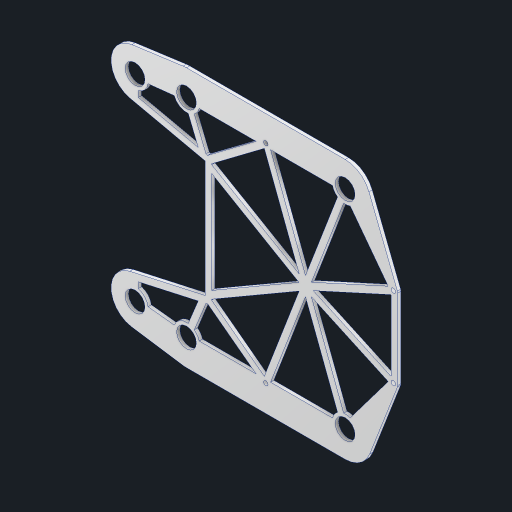
# Autodesk Inventor part: OUTK_002_ShotPlateNoReceptacle
Saved by Autodesk Inventor 2024.2 (Build 282272000, 272)
## iProperties
Created: 2024-11-24
Part Number: OUTK_002_ShotPlateNoReceptacle
Material: Aluminum 6061
Document SubType Name: Modeling
Designer: Bryan
Density: 2.7 g/cm^3
Appearance: Aluminum - Flat
Mass: 1558.28 g
Surface Area: 2532.23 cm^2
Volume: 577.142 cm^3
Author: Bryan
Autodesk Inventor part; units mm, degrees
ref_plane "YZ Plane" through (0, 0, 0) normal (1, 0, 0) x (0, 1, 0)
ref_plane "XZ Plane" through (0, 0, 0) normal (0, 1, 0) x (-1, 0, 0)
ref_plane "XY Plane" through (0, 0, 0) normal (0, 0, 1) x (1, 0, 0)
sketch "Sketch1" plane through (0, 0, 0) normal (0, 0, 1) x (1, 0, 0)
  circle A0 centre (0, 142.875) radius 63.5 construction
  circle A1 centre (0, 142.875) radius 25.4 construction
  circle A2 centre (0, -142.875) radius 25.4 construction
  circle A3 centre (0, -142.875) radius 63.5 construction
  line L0 (0, 79.375) -> (0, 79.375) construction
  line L1 (0, -79.375) -> (0, -79.375) construction
  line L2 (0, 0) -> (228.6, 0) construction
  line L3 (0, 142.875) -> (304.8, 142.875) construction
  line L4 (304.8, 142.875) -> (304.8, -142.875) construction
  line L5 (304.8, -142.875) -> (0, -142.875) construction
  circle A4 centre (228.6, 0) radius 127 construction
  circle A5 centre (0, 142.875) radius 14.2875
  circle A6 centre (0, -142.875) radius 14.2875
  circle A7 centre (0, 142.875) radius 34.925 construction
  circle A8 centre (0, -142.875) radius 34.925 construction
  circle A9 centre (74.585, -150.8125) radius 22.225 construction
  circle A10 centre (74.585, -150.8125) radius 33.3375 construction
  circle A11 centre (74.585, -150.8125) radius 11.1125 construction
  line L6 (74.585, -139.7) -> (74.585, -128.5875) construction
  line L7 (74.585, -117.475) -> (74.585, -128.5875) construction
  circle A12 centre (304.8, -150.8125) radius 33.3375 construction
  circle A13 centre (304.8, -150.8125) radius 14.2875
  circle A14 centre (374.65, 58.0572) radius 6.35 construction
  circle A15 centre (374.65, -58.0572) radius 6.35 construction
  line L8 (304.8, 150.8125) -> (374.65, 58.0572) construction
  line L9 (374.65, 58.0572) -> (374.65, -58.0572) construction
  line L10 (374.65, -58.0572) -> (304.8, -150.8125) construction
  line L11 (-118.745, 84.5312) -> (101.6, 84.5312) construction
  line L12 (101.6, 84.5312) -> (101.6, -84.5312) construction
  line L13 (101.6, -84.5312) -> (-118.745, -84.5312) construction
  line L14 (-118.745, -84.5312) -> (-118.745, 84.5312) construction
  line L15 (0, 142.875) -> (0, 84.5312) construction
  line L16 (0, -84.5312) -> (0, -142.875) construction
  circle A16 centre (74.585, -150.8125) radius 14.2875
  line L17 (74.585, -117.475) -> (304.8, -117.475) construction
  circle A17 centre (74.585, 0) radius 127 construction
  circle A18 centre (0, 0) radius 127 construction
  circle A19 centre (0, 142.875) radius 6.35 construction
  circle A20 centre (74.585, 150.8125) radius 33.3375 construction
  circle A21 centre (304.8, 150.8125) radius 33.3375 construction
  circle A22 centre (304.8, 150.8125) radius 14.2875
  circle A23 centre (74.585, 150.8125) radius 14.2875
  circle A24 centre (74.585, 150.8125) radius 37.1475 construction
  circle A25 centre (304.8, 150.8125) radius 37.1475 construction
  circle A26 centre (304.8, -150.8125) radius 38.1 construction
  circle A27 centre (74.585, -150.8125) radius 38.1 construction
  line L18 (-4.7233, 177.4791) -> (69.5611, 187.6187)
  line L19 (74.585, 187.96) -> (304.8, 187.96)
  line L20 (339.3386, 164.488) -> (380.554, 60.3949)
  line L21 (381, 58.0572) -> (381, -58.0572)
  line L22 (68.953, -188.4939) -> (-5.1627, -177.4163)
  line L23 (220.4162, -245.7989) -> (237.7908, -293.5353) construction
  line L24 (237.7908, -293.5353) -> (381, -241.4114) construction
  line L25 (381, -241.4114) -> (363.6254, -193.675) construction
  line L26 (363.6254, -193.675) -> (220.4162, -245.7989) construction
  line L27 (-7.573, -108.7809) -> (101.6, -84.5312)
  line L28 (-7.573, 108.7809) -> (101.6, 84.5312)
  line L29 (101.6, 84.5312) -> (101.6, -84.5312)
  circle A28 centre (238.125, 0) radius 127
  line L30 (101.6, 0) -> (111.125, 0)
  line L31 (374.65, 0) -> (365.125, 0)
  circle A29 centre (220.4162, -245.7989) radius 3.2512 construction
  circle A30 centre (268.1526, -228.4242) radius 3.2512 construction
  circle A31 centre (315.889, -211.0496) radius 3.2512 construction
  circle A32 centre (363.6254, -193.675) radius 3.2512 construction
  circle A33 centre (237.7908, -293.5353) radius 3.2512 construction
  circle A34 centre (285.5272, -276.1606) radius 3.2512 construction
  circle A35 centre (333.2636, -258.786) radius 3.2512 construction
  circle A36 centre (381, -241.4114) radius 3.2512 construction
  line L32 (74.585, -188.9125) -> (304.8, -188.9125)
  line L33 (380.5737, -60.3445) -> (340.3424, -164.5364)
  arc A37 (-4.7233, 177.4791) -> (-7.573, 108.7809) centre (0, 142.875) ccw
  arc A38 (74.585, 187.96) -> (69.5611, 187.6187) centre (74.585, 150.8125) ccw
  arc A39 (339.3386, 164.488) -> (304.8, 187.96) centre (304.8, 150.8125) ccw
  arc A40 (381, 58.0572) -> (380.554, 60.3949) centre (374.65, 58.0572) ccw
  arc A41 (380.5737, -60.3445) -> (381, -58.0572) centre (374.65, -58.0572) ccw
  arc A42 (304.8, -188.9125) -> (340.3424, -164.5364) centre (304.8, -150.8125) ccw
  arc A43 (68.953, -188.4939) -> (74.585, -188.9125) centre (74.585, -150.8125) ccw
  arc A44 (-7.573, -108.7809) -> (-5.1627, -177.4163) centre (0, -142.875) ccw
  circle A45 centre (374.65, 58.0572) radius 3.2512
  circle A46 centre (374.65, -58.0572) radius 3.2512
  circle A47 centre (189.6925, 150.8125) radius 3.2512
  line L34 (74.585, 150.8125) -> (189.6925, 150.8125) construction
  line L35 (189.6925, 150.8125) -> (304.8, 150.8125) construction
  circle A48 centre (189.6925, -150.8125) radius 3.2512
  line L36 (74.585, -150.8125) -> (304.8, -150.8125) construction
  point P0 (0, 117.475)
  point P1 (0, -117.475)
  point P2 (304.8, 0)
  point P3 (228.6, -127)
  point P4 (228.6, -127)
  point P5 (355.6, 0)
  point P6 (0, 127)
  point P7 (0, 117.475)
  point P8 (0, 136.525)
  dimension "d1" = 50.8
  dimension "d16" = 44.45
  dimension "d20" = 22.225
  dimension "d33" = 12.7
  dimension "d0" = 127
  dimension "d3" = 285.75
  dimension "d4" = 254
  dimension "d6" = 158.75
  dimension "d7" = 234.95
  dimension "d11" = 28.575
  dimension "d12" = 28.575
  dimension "d13" = 69.85
  dimension "d14" = 69.85
  dimension "d19" = 76.2
  dimension "d22" = 304.8
  dimension "d24" = 28.575
  dimension "d26" = 12.7
  dimension "d27" = 12.7
  dimension "d28" = 19.05
  dimension "d29" = 220.345
  dimension "d30" = 169.0624
  dimension "d31" = 9.525
  dimension "d32" = 75.0062
  dimension "d34" = 9.525
  dimension "d35" = 19.05
  dimension "d37" = 3.81
  dimension "d38" = 3.81
  dimension "d39" = 4.7625
  dimension "d40" = 4.7625
  dimension "d43" = 20
  dimension "d44" = 6.5024
  dimension "d47" = 50.8
  dimension "d50" = 50.8
  dimension "d53" = 50.8
  dimension "d56" = 6.5024
  dimension "d57" = 6.5024
  dimension "d58" = 6.5024
  dimension "d105" = 230.215
  constraints: 74 end point, 41 centre point, 41 point on circle, 24 tangent, 21 coincident, 16 vertical alignment, 11 horizontal, 7 perpendicular, 7 point on line, 6 concentric, 6 equal length, 6 symmetric about line, 4 equal radius, 4 vertical, 3 horizontal alignment, 3 midpoint, 2 parallel, 41 other
  measures "d0" diameter of A0
  measures "d3" distance between parallel lines of L5 L3
  measures "d4" diameter of A4
  measures "d6" distance of L1.start L0.start
  measures "d7" distance of point (0, -117.475) point (0, 117.475)
  measures "d11" diameter of A5
  measures "d12" diameter of A6
  measures "d13" diameter of A7
  measures "d14" diameter of A8
  measures "d19" distance of point (304.8, 0) L2.end
  measures "d22" distance of L3.end A0.centre
  measures "d24" diameter of A13
  measures "d26" diameter of A14
  measures "d27" diameter of A15
  measures "d28" distance from line of L9 point (355.6, 0)
  measures "d29" distance of L12.end L13.end
  measures "d30" distance of L11.end L12.end
  measures "d31" distance from line of L17 A4.start
  measures "d32" distance of point (74.585, -150.812) point (0, -142.875)
  measures "d34" distance of point (0, 117.475) point (0, 127)
  measures "d35" distance of point (0, 117.475) point (0, 136.525)
  measures "d37" radial gap between concentric circles of A20 A24
  measures "d38" radial gap between concentric circles of A21 A25
  measures "d43" angle of L26 L5
  measures "d44" diameter of A29
  measures "d47" distance of A29.centre A30.centre
  measures "d50" distance of A29.centre A33.centre
  measures "d53" distance from line of L25.end L5
  measures "d56" diameter of A45
  measures "d57" diameter of A46
  measures "d58" diameter of A47
  measures "d105" distance of L36.start L36.end
extrude "Extrusion1" add sketch "Sketch1" along normal mid plane 4.7625 contours L18 A38 L19 A39 L20 A40 L21 A41 L33 A42 L32 A43 L22 A44 L27 L29 L28 A37 | A28
sketch "Sketch2" plane through (0, 0, -2.3813) normal (0, 0, -1) x (-1, 0, 0)
  line L0 (7.573, -108.7809) -> (-101.6, -84.5312) projected
  line L1 (-101.6, -84.5312) -> (-101.6, 84.5312) projected
  line L2 (-101.6, 84.5312) -> (7.573, 108.7809) projected
  arc A0 (7.573, 108.7809) -> (4.7233, 177.4791) centre (0, 142.875) ccw projected
  line L3 (4.7233, 177.4791) -> (-69.5611, 187.6187) projected
  arc A1 (-69.5611, 187.6187) -> (-74.585, 187.96) centre (-74.585, 150.8125) ccw projected
  line L4 (-74.585, 187.96) -> (-304.8, 187.96) projected
  arc A2 (-304.8, 187.96) -> (-339.3386, 164.488) centre (-304.8, 150.8125) ccw projected
  line L5 (-339.3386, 164.488) -> (-380.554, 60.3949) projected
  arc A3 (-380.554, 60.3949) -> (-381, 58.0572) centre (-374.65, 58.0572) ccw projected
  line L6 (-381, 58.0572) -> (-381, -58.0572) projected
  arc A4 (-381, -58.0572) -> (-380.5737, -60.3445) centre (-374.65, -58.0572) ccw projected
  line L7 (-380.5737, -60.3445) -> (-340.3424, -164.5364) projected
  arc A5 (-340.3424, -164.5364) -> (-304.8, -188.9125) centre (-304.8, -150.8125) ccw projected
  line L8 (-304.8, -188.9125) -> (-74.585, -188.9125) projected
  arc A6 (-74.585, -188.9125) -> (-68.953, -188.4939) centre (-74.585, -150.8125) ccw projected
  line L9 (-68.953, -188.4939) -> (5.1627, -177.4163) projected
  arc A7 (5.1627, -177.4163) -> (7.573, -108.7809) centre (0, -142.875) ccw projected
  circle A8 centre (-74.585, -150.8125) radius 14.2875 projected
  circle A9 centre (-74.585, 150.8125) radius 14.2875 projected
  circle A10 centre (-189.6925, 150.8125) radius 3.2512 projected
  circle A11 centre (-189.6925, -150.8125) radius 3.2512 projected
  circle A12 centre (-374.65, -58.0572) radius 3.2512 projected
  circle A13 centre (-374.65, 58.0572) radius 3.2512 projected
  circle A14 centre (-304.8, 150.8125) radius 14.2875 projected
  circle A15 centre (-304.8, -150.8125) radius 14.2875 projected
  circle A16 centre (0, -142.875) radius 14.2875 projected
  circle A17 centre (0, 142.875) radius 14.2875 projected
  line L10 (-106.3625, -88.3519) -> (6.5404, -113.4301)
  arc A18 (4.4587, -172.7061) -> (6.5404, -113.4301) centre (0, -142.875) ccw
  line L11 (4.4587, -172.7061) -> (-69.657, -183.7838)
  arc A19 (-74.585, -184.15) -> (-69.657, -183.7838) centre (-74.585, -150.8125) ccw
  line L12 (-74.585, -184.15) -> (-304.8, -184.15)
  arc A20 (-335.8996, -162.8209) -> (-304.8, -184.15) centre (-304.8, -150.8125) ccw
  line L13 (-335.8996, -162.8209) -> (-376.1309, -58.6291)
  arc A21 (-376.2375, -58.0572) -> (-376.1309, -58.6291) centre (-374.65, -58.0572) ccw
  line L14 (-376.2375, -58.0572) -> (-376.2375, 58.0572)
  arc A22 (-376.126, 58.6416) -> (-376.2375, 58.0572) centre (-374.65, 58.0572) ccw
  line L15 (-376.126, 58.6416) -> (-334.9106, 162.7347)
  arc A23 (-304.8, 183.1975) -> (-334.9106, 162.7347) centre (-304.8, 150.8125) ccw
  line L16 (-304.8, 183.1975) -> (-74.585, 183.1975)
  arc A24 (-70.2052, 182.9) -> (-74.585, 183.1975) centre (-74.585, 150.8125) ccw
  line L17 (-70.2052, 182.9) -> (4.0793, 172.7604)
  arc A25 (6.5404, 113.4301) -> (4.0793, 172.7604) centre (0, 142.875) ccw
  line L18 (6.5404, 113.4301) -> (-106.3625, 88.3519)
  line L19 (-106.3625, 88.3519) -> (-106.3625, -88.3519)
  circle A26 centre (-74.585, 150.8125) radius 19.05
  circle A27 centre (0, 142.875) radius 19.05
  circle A28 centre (-189.6925, 150.8125) radius 8.0137
  circle A29 centre (-304.8, 150.8125) radius 19.05
  circle A30 centre (-374.65, 58.0572) radius 8.0137
  circle A31 centre (-374.65, -58.0572) radius 8.0137
  circle A32 centre (-304.8, -150.8125) radius 19.05
  circle A33 centre (-189.6925, -150.8125) radius 8.0137
  circle A34 centre (-74.585, -150.8125) radius 19.05
  circle A35 centre (0, -142.875) radius 19.05
  line L20 (0, -142.875) -> (-74.585, -150.8125)
  line L21 (-74.585, -150.8125) -> (-71.7613, -188.8077)
  line L22 (-74.585, -150.8125) -> (-101.6, -84.5312)
  line L23 (-74.585, -150.8125) -> (-189.6925, -150.8125)
  line L24 (-189.6925, -150.8125) -> (-189.6925, -188.9125)
  line L25 (-189.6925, -150.8125) -> (-304.8, -150.8125)
  line L26 (-304.8, -150.8125) -> (-326.3491, -182.233)
  line L27 (-101.6, -84.5312) -> (-247.2463, 0)
  line L28 (-247.2463, 0) -> (-189.6925, -150.8125)
  line L29 (-304.8, -150.8125) -> (-247.2463, 0)
  line L30 (-247.2463, 0) -> (-374.65, -58.0572)
  line L31 (-247.2463, 0) -> (-374.65, 58.0572)
  line L32 (-374.65, 58.0572) -> (-304.8, 150.8125)
  line L33 (-304.8, 150.8125) -> (-189.6925, 150.8125)
  line L34 (-189.6925, 150.8125) -> (-74.585, 150.8125)
  line L35 (-74.585, 150.8125) -> (0, 142.875)
  line L36 (-101.6, -84.5312) -> (-189.6925, -150.8125)
  line L37 (-304.8, -150.8125) -> (-374.65, -58.0572)
  line L38 (-101.6, 84.5312) -> (-74.585, 150.8125)
  line L39 (-101.6, 84.5312) -> (-189.6925, 150.8125)
  line L40 (-101.6, 84.5312) -> (-247.2463, 0)
  line L41 (-247.2463, 0) -> (-189.6925, 150.8125)
  line L42 (-247.2463, 0) -> (-304.8, 150.8125)
  line L43 (-4.7625, -138.5924) -> (-75.089, -146.0767)
  line L44 (-70.1748, -149.015) -> (-99.7912, -76.351)
  line L45 (0, -142.875) -> (0, -111.9774)
  line L46 (-4.7625, -110.9195) -> (-4.7625, -138.5924)
  line L47 (0, 142.875) -> (0, 111.9774)
  line L48 (-99.7912, 76.351) -> (-70.1748, 149.015)
  line L49 (-108.6117, 79.9461) -> (-78.9953, 152.61)
  line L50 (-189.6925, 146.05) -> (-74.0459, 146.05)
  line L51 (-95.603, 85.979) -> (-186.8292, 154.6181)
  line L52 (-110.2034, 85.0444) -> (-254.722, 1.1677)
  line L53 (-101.3297, 78.3678) -> (-192.5559, 147.0069)
  line L54 (-241.8175, 0.868) -> (-184.3245, 151.5213)
  line L55 (-250.5386, 4.7303) -> (-193.0456, 155.3836)
  line L56 (-304.8, 146.05) -> (-189.6925, 146.05)
  line L57 (-244.0343, 4.9409) -> (-303.5695, 160.9454)
  line L58 (-253.0929, 1.963) -> (-312.6281, 157.9675)
  line L59 (-299.7883, 149.5508) -> (-367.277, 59.9311)
  line L60 (-367.277, 59.9311) -> (-252.4677, 7.6131)
  line L61 (-256.6012, -0.9707) -> (-382.023, 56.1834)
  line L62 (-382.023, 56.1834) -> (-307.3971, 155.2807)
  line L63 (-257.3107, 0.6474) -> (-382.023, -56.1834)
  line L64 (-382.023, -56.1834) -> (-307.3971, -155.2807)
  line L65 (-253.1772, -7.9364) -> (-367.277, -59.9311)
  line L66 (-367.277, -59.9311) -> (-299.7883, -149.5508)
  line L67 (-313.266, -159.6391) -> (-253.7308, -3.6346)
  line L68 (-251.9417, -1.0535) -> (-194.4487, -151.7068)
  line L69 (-243.2206, 2.8088) -> (-185.7277, -147.8445)
  line L70 (-304.2074, -162.617) -> (-244.6722, -6.6125)
  line L71 (-110.2034, -85.0444) -> (-254.722, -1.1677)
  line L72 (-106.3625, -76.2606) -> (-250.178, 7.2081)
  line L73 (-106.3625, 76.2606) -> (-250.178, -7.2081)
  line L74 (-78.9953, -152.61) -> (-108.6117, -79.9461)
  line L75 (-103.1152, -79.7113) -> (-194.3414, -148.3504)
  line L76 (-95.603, -85.979) -> (-186.8292, -154.6181)
  line L77 (-74.585, -146.05) -> (-190.2316, -146.05)
  line L78 (-189.6925, -146.05) -> (-305.3391, -146.05)
  line L79 (-75.089, 146.0767) -> (-4.7625, 138.5924)
  line L80 (-4.7625, 138.5924) -> (-4.7625, 110.9195)
  arc A36 (-376.2375, -6.35) -> (-371.3291, -6.2352) centre (-373.782, -6.35) ccw
  arc A37 (-371.3291, 6.2352) -> (-376.2375, 6.35) centre (-373.782, 6.35) ccw
  line L81 (-247.2463, 0) -> (-365.125, 0)
  line L82 (-111.125, 92.1726) -> (5.5077, 118.0793)
  arc A38 (5.5077, 118.0793) -> (3.4352, 168.0416) centre (0, 142.875) ccw
  line L83 (3.4352, 168.0416) -> (-70.8493, 178.1812)
  arc A39 (-70.8493, 178.1812) -> (-74.585, 178.435) centre (-74.585, 150.8125) ccw
  line L84 (-74.585, 178.435) -> (-304.8, 178.435)
  arc A40 (-304.8, 178.435) -> (-330.4826, 160.9815) centre (-304.8, 150.8125) ccw
  line L85 (-330.4826, 160.9815) -> (-371.475, 57.4515)
  line L86 (-371.475, 57.4515) -> (-371.475, -57.4655)
  line L87 (-371.475, -57.4655) -> (-331.4568, -161.1054)
  arc A41 (-331.4568, -161.1054) -> (-304.8, -179.3875) centre (-304.8, -150.8125) ccw
  line L88 (-304.8, -179.3875) -> (-74.585, -179.3875)
  arc A42 (-74.585, -179.3875) -> (-70.361, -179.0736) centre (-74.585, -150.8125) ccw
  line L89 (-70.361, -179.0736) -> (3.7547, -167.996)
  arc A43 (3.7547, -167.996) -> (5.5077, -118.0793) centre (0, -142.875) ccw
  line L90 (5.5077, -118.0793) -> (-111.125, -92.1726)
  line L91 (-111.125, -92.1726) -> (-111.125, 92.1726)
  point P0 (0, 0)
  point P1 (-247.2463, 146.05)
  point P2 (-376.2375, 0)
  point P3 (-4.7625, -124.4299)
  point P4 (-93.7588, -91.1515)
  point P5 (-77.1366, -131.9342)
  point P6 (-56.7475, -144.1248)
  point P7 (-18.8455, -140.0912)
  point P8 (-175.4415, -146.05)
  point P9 (-93.0301, -146.05)
  point P10 (-85.9571, -135.5292)
  point P11 (-103.6768, -92.0538)
  point P12 (-237.7586, 0)
  point P13 (-187.4058, -143.132)
  point P14 (-237.9992, -10.8734)
  point P15 (-187.5409, -143.093)
  point P16 (-286.3549, -146.05)
  point P17 (-196.6075, -146.05)
  point P18 (-247.2463, -13.3574)
  point P19 (-293.774, -135.2777)
  point P20 (-302.673, -131.8816)
  point P21 (-255.8346, -9.1474)
  point P22 (-366.8104, -59.7184)
  point P23 (-366.9685, -60.3407)
  point P24 (-312.0914, -133.2131)
  point P25 (-370.7601, -51.0509)
  point P26 (-258.7313, 0)
  point P27 (-370.7601, 51.0509)
  point P28 (-376.2375, 50.2023)
  point P29 (-376.2375, -50.2023)
  point P30 (-366.8104, 59.7184)
  point P31 (-255.8346, 9.1474)
  point P32 (-302.673, 131.8816)
  point P33 (-312.0914, 133.2131)
  point P34 (-366.9685, 60.3407)
  point P35 (-293.774, 135.2777)
  point P36 (-247.2463, 13.3574)
  point P37 (-196.6075, 146.05)
  point P38 (-286.3549, 146.05)
  point P39 (-187.5409, 143.093)
  point P40 (-237.9992, 10.8734)
  point P41 (-187.4058, 143.132)
  point P42 (-175.4415, 146.05)
  point P43 (-103.6768, 92.0538)
  point P44 (-85.9571, 135.5292)
  point P45 (-93.0301, 146.05)
  point P46 (-4.7625, 124.4299)
  point P47 (-18.8455, 140.0912)
  point P48 (-56.7475, 144.1248)
  point P49 (-77.1366, 131.9342)
  point P50 (-93.7588, 91.1515)
  point P51 (-91.5725, 96.5157)
  point P52 (-4.7625, 115.7981)
  point P53 (-105.4964, 93.4229)
  point P54 (-102.8821, 94.0036)
  point P55 (-111.125, 84.5095)
  point P56 (-111.125, 85.7379)
  point P57 (-371.475, -50.6993)
  point P58 (-371.475, 50.6993)
  point P59 (-111.125, -85.7379)
  point P60 (-111.125, -84.5095)
  point P61 (-111.125, -73.4965)
  point P62 (-111.125, 73.4965)
  point P63 (-102.8821, -94.0036)
  point P64 (-105.4964, -93.4229)
  point P65 (-4.7625, -115.7981)
  point P66 (-91.5725, -96.5157)
  dimension "d59" = 4.7625
  dimension "d61" = 4.7625
  dimension "d62" = 4.7625
  dimension "d63" = 4.7625
  dimension "d64" = 4.7625
  dimension "d65" = 4.7625
  dimension "d66" = 4.7625
  dimension "d67" = 4.7625
  dimension "d68" = 4.7625
  dimension "d69" = 4.7625
  dimension "d70" = 4.7625
  dimension "d71" = 4.7625
  dimension "d72" = 4.7625
  dimension "d73" = 4.7625
  dimension "d75" = 4.7625
  dimension "d76" = 4.7625
  dimension "d77" = 4.7625
  dimension "d78" = 4.7625
  dimension "d79" = 4.7625
  dimension "d80" = 4.7625
  dimension "d81" = 4.7625
  dimension "d82" = 4.7625
  dimension "d83" = 4.7625
  dimension "d84" = 4.7625
  dimension "d85" = 4.7625
  dimension "d86" = 4.7625
  dimension "d87" = 4.7625
  dimension "d88" = 4.7625
  dimension "d89" = 4.7625
  dimension "d90" = 4.7625
  dimension "d91" = 4.7625
  dimension "d92" = 4.7625
  dimension "d93" = 4.7625
  dimension "d94" = 4.7625
  dimension "d95" = 4.7625
  dimension "d96" = 4.7625
  dimension "d97" = 4.7625
  dimension "d98" = 4.7625
  dimension "d99" = 4.7625
  dimension "d100" = 4.7625
  dimension "d101" = 4.7625
  dimension "d102" = 4.7625
  dimension "d103" = 4.7625
  dimension "d104" = 12.7
  dimension "d108" = 4.7625
  constraints: 164 end point, 34 point on circle, 26 centre point, 25 parallel, 10 point on line, 5 horizontal, 3 midpoint, 3 vertical alignment, 2 tangent, 2 vertical, 1 horizontal alignment, 1 symmetric about line, 36 other
  measures "d59" distance between parallel lines of L0 L10
  measures "d61" radial gap between concentric circles of A9 A26
  measures "d62" radial gap between concentric circles of A17 A27
  measures "d63" radial gap between concentric circles of A10 A28
  measures "d64" radial gap between concentric circles of A14 A29
  measures "d65" radial gap between concentric circles of A13 A30
  measures "d66" radial gap between concentric circles of A12 A31
  measures "d67" radial gap between concentric circles of A15 A32
  measures "d68" radial gap between concentric circles of A11 A33
  measures "d69" radial gap between concentric circles of A8 A34
  measures "d70" radial gap between concentric circles of A16 A35
  measures "d71" distance between parallel lines of L20 L43
  measures "d72" distance between parallel lines of L22 L44
  measures "d73" distance between parallel lines of L45 L46
  measures "d75" distance between parallel lines of L38 L48
  measures "d76" distance between parallel lines of L38 L49
  measures "d77" distance between parallel lines of L34 L50
  measures "d78" distance between parallel lines of L39 L51
  measures "d79" distance between parallel lines of L40 L52
  measures "d80" distance between parallel lines of L39 L53
  measures "d81" distance between parallel lines of L41 L54
  measures "d82" distance between parallel lines of L41 L55
  measures "d83" distance between parallel lines of L33 L56
  measures "d84" distance between parallel lines of L42 L57
  measures "d85" distance between parallel lines of L42 L58
  measures "d86" distance between parallel lines of L32 L59
  measures "d87" distance between parallel lines of L31 L61
  measures "d88" distance between parallel lines of L30 L63
  measures "d89" distance between parallel lines of L30 L65
  measures "d90" distance between parallel lines of L29 L67
  measures "d91" distance between parallel lines of L28 L68
  measures "d92" distance between parallel lines of L28 L69
  measures "d93" distance between parallel lines of L29 L70
  measures "d94" distance between parallel lines of L27 L71
  measures "d95" distance between parallel lines of L27 L72
  measures "d96" distance between parallel lines of L40 L73
  measures "d97" distance between parallel lines of L22 L74
  measures "d98" distance between parallel lines of L36 L75
  measures "d99" distance between parallel lines of L36 L76
  measures "d100" distance between parallel lines of L23 L77
  measures "d101" distance between parallel lines of L25 L78
  measures "d102" distance between parallel lines of L35 L79
  measures "d103" distance between parallel lines of L47 L80
  measures "d104" distance of A37.centre A36.centre
  measures "d108" distance between parallel lines of L18 L82
extrude "Not Final Pocketing" cut sketch "Sketch2" against normal blind 25.4 contours L90 L46 A35 L43 A34 L44 | L74 A34 L77 L76 L90 | L72 L73 L91 | L75 A33 L69 L71 L91 | L48 A26 L79 A27 L80 L82 | L82 L51 L50 A26 L49 | L91 L52 L54 A28 L53 | L63 A31 L86 A30 L61 | L68 L78 A32 L70 | L57 A29 L56 L55 | L60 A30 L59 A29 L58 | L66 A31 L65 L67 A32
body "Solid1"
